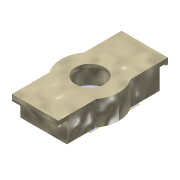
# Autodesk Inventor part: ECoG_holder
Saved by Autodesk Inventor 2014 (Build 180170000, 170)
## iProperties
Created: 2016-07-07
Part Number: ECoG_holder
Material: Generic
Document SubType Name: Modeling
Designer: Camilo
Density: 1 g/cm^3
Appearance: Fine - Cream
Author: Camilo
Autodesk Inventor part; units mm, degrees
ref_plane "YZ Plane" through (0, 0, 0) normal (1, 0, 0) x (0, 1, 0)
ref_plane "XZ Plane" through (0, 0, 0) normal (0, 1, 0) x (-1, 0, 0)
ref_plane "XY Plane" through (0, 0, 0) normal (0, 0, 1) x (1, 0, 0)
sketch "Sketch1" plane through (0, 0, 0) normal (0, 0, 1) x (1, 0, 0)
  circle A0 centre (0, 0) radius 10.575 projected
  circle A1 centre (0, 0) radius 10.675
  point P0 (0, 0)
  dimension "d0" = 0.1
  constraints: 1 centre point, 1 coincident
  measures "d0" radial gap between concentric circles of A1 A0
extrude "Extrusion1" add sketch "Sketch1" along normal blind 1.5 contours A0 | A1
sketch "Sketch2" plane through (0, 0, 1.5) normal (0, 0, 1) x (1, 0, 0)
  circle A0 centre (0, 0) radius 10.675 projected
  circle A1 centre (0, 0) radius 13.675
  dimension "d3" = 3
  constraints: 1 centre point, 1 coincident
  measures "d3" radial gap between concentric circles of A1 A0
extrude "Extrusion2" add sketch "Sketch2" against normal blind 7
sketch "Sketch4" plane through (0, 0, 1.5) normal (0, 0, 1) x (1, 0, 0)
  line L0 (-9, -24.94) -> (9, -24.94) construction
  line L1 (9, -24.94) -> (9, -6.94) construction
  line L2 (9, -6.94) -> (-9, -6.94) construction
  line L3 (-9, -6.94) -> (-9, -24.94) construction
  line L4 (-11, -25.94) -> (11, -25.94)
  line L5 (11, -25.94) -> (11, -6.4004)
  line L6 (-11, -6.4004) -> (-11, -25.94)
  line L7 (-11, -6.4004) -> (11, -6.4004)
  circle A0 centre (0, 0) radius 10.575 projected
  circle A1 centre (0, 0) radius 10.575
  circle A2 centre (0, 0) radius 10.575 projected
  circle A3 centre (0, 0) radius 10.575
  circle A4 centre (0, 0) radius 10.675 projected
  arc A5 (-8.5435, -6.4004) -> (8.5435, -6.4004) centre (0, 1.4092) ccw
  dimension "d8" = 2
  dimension "d9" = 2
  dimension "d10" = 1
  constraints: 8 end point, 4 point on circle, 3 centre point, 2 point on line, 4 other
  measures "d8" distance between parallel lines of L6 L3
  measures "d9" distance between parallel lines of L5 L1
  measures "d10" distance between parallel lines of L0 L4
extrude "Extrusion4" add sketch "Sketch4" against normal up to surface (7 mm away) contours L6 L7 A4 L5 L4 | A5 A0 A4 | L7 A0 A5 | A5 A0 L7 | L7 A0 A5 | A5 A0
sketch "Sketch5" plane through (0, 0, 1.5) normal (0, 0, 1) x (1, 0, 0)
  line L0 (-11, -8.1244) -> (-11, -25.94) construction
  line L1 (-11, -25.94) -> (11, -25.94) construction
  line L2 (11, -25.94) -> (11, -8.1244) construction
  line L3 (-9, -24.94) -> (9, -24.94) construction
  line L4 (9, -24.94) -> (9, -6.94) construction
  line L5 (9, -6.94) -> (-9, -6.94) construction
  line L6 (-9, -6.94) -> (-9, -24.94) construction
  line L7 (-9.25, -18.44) -> (-11, -18.44)
  line L8 (-11, -18.44) -> (-11, -25.94)
  line L9 (9.25, -18.44) -> (11, -18.44)
  line L10 (11, -18.44) -> (11, -25.94)
  line L11 (-9.25, -18.44) -> (-9.25, -25.04)
  line L12 (-9.25, -25.04) -> (-8, -25.04)
  line L13 (-8, -25.04) -> (-8, -25.94)
  line L14 (9.25, -18.44) -> (9.25, -25.04)
  line L15 (9.25, -25.04) -> (8, -25.04)
  line L16 (8, -25.04) -> (8, -25.94)
  line L17 (-11, -25.94) -> (-8, -25.94)
  line L18 (8, -25.94) -> (11, -25.94)
  dimension "d14" = 7.5
  dimension "d15" = 0.25
  dimension "d16" = 0.1
  dimension "d17" = 1
  dimension "d18" = 0.25
  dimension "d19" = 0.1
  dimension "d20" = 1
  constraints: 24 end point, 2 point on line
  measures "d14" distance between parallel lines of L1 L9
  measures "d15" distance between parallel lines of L11 L6
  measures "d16" distance between parallel lines of L12 L3
  measures "d17" distance between parallel lines of L13 L6
  measures "d18" distance between parallel lines of L14 L4
  measures "d19" distance between parallel lines of L15 L3
  measures "d20" distance between parallel lines of L16 L4
extrude "Extrusion5" [suppressed]
sketch "Sketch6" plane through (0, 0, 2) normal (0, 0, 1) x (1, 0, 0)
  line L0 (-11, -18.44) -> (-11, -25.94) construction
  line L1 (-11, -25.94) -> (-8, -25.94) construction
  line L2 (-8, -25.94) -> (-8, -25.04) construction
  line L3 (-8, -25.04) -> (-9.25, -25.04) construction
  line L4 (-9.25, -25.04) -> (-9.25, -18.44) construction
  line L5 (-9.25, -18.44) -> (-11, -18.44) construction
  line L6 (-8, -18.44) -> (-11, -18.44)
  line L7 (-11, -18.44) -> (-11, -25.94)
  line L8 (-11, -25.94) -> (-8, -25.94)
  line L9 (-8, -25.94) -> (-8, -18.44)
  line L10 (8, -18.44) -> (11, -18.44)
  line L11 (11, -18.44) -> (11, -25.94)
  line L12 (11, -25.94) -> (8, -25.94)
  line L13 (8, -25.94) -> (8, -18.44)
  point P0 (0, 0)
  constraints: 16 end point
extrude "Extrusion6" [suppressed]
sketch "Sketch8" plane through (-11, -25.94, -5.5) normal (0, -1, 0) x (1, 0, 0)
  line L0 (0, 7) -> (22, 7) construction
  line L1 (0, 7) -> (0, 0) construction
  line L2 (22, 0) -> (0, 0)
  line L3 (0, 0) -> (0, 5)
  line L4 (0, 5) -> (22, 5)
  line L5 (22, 5) -> (22, 0)
  point P0 (19, 7)
  point P1 (3, 7)
  point P2 (0, 7.5)
  point P3 (11, 5.5)
  dimension "d27" = 2
  constraints: 8 end point, 1 point on line
  measures "d27" distance between parallel lines of L0 L4
extrude "Extrusion8" cut sketch "Sketch8" against normal blind 4
mirror "Mirror1" about plane through (0, 0, 0) normal (0, 1, 0) of "Extrusion8", "Extrusion4"
sketch "Sketch3" plane through (0, 0, 1.5) normal (0, 0, 1) x (1, 0, 0)
  circle A0 centre (0, 0) radius 6.94 projected
extrude "Extrusion3" cut sketch "Sketch3" against normal through all
sketch "Sketch7" plane through (0, 0, 0) normal (0, 0, -1) x (-1, 0, 0)
  arc A0 (8.5435, -6.4004) -> (-8.5435, -6.4004) centre (0, 0) ccw construction
  circle A1 centre (0, 0) radius 10.95
  dimension "d30" = 0.275
  constraints: 1 centre point, 1 coincident
  measures "d30" radial gap between concentric circles of A0 A1
extrude "Extrusion7" cut sketch "Sketch7" along normal up to surface (5.5 mm away)
sketch "Sketch9" plane through (11, 25.94, -0.5) normal (0, 0, -1) x (-1, 0, 0)
  line L0 (22, 0) -> (22, -4) construction
  line L1 (0, 0) -> (22, 0)
  line L2 (22, 0) -> (22, -1)
  line L3 (22, -1) -> (0, -1)
  line L4 (0, -1) -> (0, 0)
  line L5 (22, -51.88) -> (0, -51.88) construction
  line L6 (22, -47.88) -> (22, -51.88) construction
  line L7 (22, -47.88) -> (0, -47.88) construction
  line L8 (0, -51.88) -> (0, -47.88) construction
  line L9 (22, -51.88) -> (0, -51.88)
  line L10 (0, -51.88) -> (0, -50.88)
  line L11 (0, -50.88) -> (22, -50.88)
  line L12 (22, -50.88) -> (22, -51.88)
  point P0 (11, -25.94)
  dimension "d31" = 1
  dimension "d32" = 1
  constraints: 16 end point, 2 point on line
  measures "d31" distance between parallel lines of L1 L3
  measures "d32" distance between parallel lines of L9 L11
extrude "Extrusion9" add sketch "Sketch9" along normal blind 0.8 draft 0.5
ref_plane "Work Plane1" through (0, 0, -10.15) normal (0, 0, -1) x (-1, 0, 0)
sketch "Sketch10" plane through (0, 0, -5.5) normal (0, 0, -1) x (-1, 0, 0)
  circle A0 centre (0, 0) radius 10.95 projected
  line L0 (11, 21.94) -> (-11, 21.94) projected
  line L1 (-11, 8.1244) -> (-11, 21.94) projected
  arc A1 (-11, 8.1244) -> (-11, -8.1244) centre (0, 0) ccw projected
  line L2 (-11, -8.1244) -> (-11, -21.94) projected
  line L3 (-11, -21.94) -> (11, -21.94) projected
  line L4 (11, -21.94) -> (11, -8.1244) projected
  arc A2 (11, -8.1244) -> (11, 8.1244) centre (0, 0) ccw projected
  line L5 (11, 21.94) -> (11, 8.1244) projected
extrude "Extrusion10" add sketch "Sketch10" along normal up to surface (4.65 mm away)
body "Solid1"
